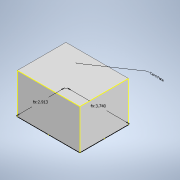
# Autodesk Inventor part: MasterPart
Saved by Autodesk Inventor 2022.2 (Build 262287010, 287A)
## iProperties
Created: 2022-07-12
Part Number: MasterPart
Material: Generic
Document SubType Name: Modeling
Designer: keaton
Density: 1 g/cm^3
Appearance: Default
d0: 3.740 in
d1: 2.913 in
d2: 2.402 in
d3: 0.00 deg
CardWidth: 74.000 mm
CardHeight: 95.000 mm
DeckThickness: 61.000 mm
PlateThickness: 4.000 mm
PuzzleWidth: 15.000 mm
Author: keaton
Autodesk Inventor part; units mm, degrees
ref_plane "YZ Plane" through (0, 0, 0) normal (1, 0, 0) x (0, 1, 0)
ref_plane "XZ Plane" through (0, 0, 0) normal (0, 1, 0) x (-1, 0, 0)
ref_plane "XY Plane" through (0, 0, 0) normal (0, 0, 1) x (1, 0, 0)
sketch "DeckFace" plane through (0, 0, 0) normal (0, 1, 0) x (-1, 0, 0)
  line L0 (-47.5, 37) -> (47.5, 37)
  line L1 (47.5, 37) -> (47.5, -37)
  line L2 (47.5, -37) -> (-47.5, -37)
  line L3 (-47.5, -37) -> (-47.5, 37)
  line L4 (-47.5, 37) -> (47.5, -37) construction
  line L5 (47.5, 37) -> (-47.5, -37) construction
  point P0 (0, 0)
  dimension "d0" = 95
  dimension "d1" = 74
  constraints: 12 end point, 2 midpoint, 2 parallel, 1 horizontal, 1 perpendicular
  measures "d0" distance of L1.end L2.end
  measures "d1" distance of L0.end L1.end
extrude "Extrusion1" add sketch "DeckFace" along normal blind 61
sketch "DeckSide" plane through (-47.5, 0, 37) normal (0, 0, 1) x (1, 0, 0)
  line L0 (0, 61) -> (95, 61) projected
  line L1 (0, 0) -> (0, 61) projected
  line L2 (0, 0) -> (95, 0) projected
  line L3 (95, 0) -> (95, 61) projected
  point P0 (47.5, 0)
sketch "DeckBottom" plane through (47.5, 0, 37) normal (1, 0, 0) x (0, 0, -1)
  line L0 (0, 0) -> (0, 61) projected
  line L1 (0, 61) -> (74, 61) projected
  line L2 (74, 0) -> (74, 61) projected
  line L3 (74, 0) -> (0, 0) projected
  point P0 (37, 0)
equation "\"d0\" = CardHeight"
equation "\"d1\" = CardWidth"
equation "\"d2\" = DeckThickness"
equation "\"CardWidth\" = 74"
equation "\"CardHeight\" = 95"
equation "\"DeckThickness\" = 61"
equation "\"PlateThickness\" = 4"
equation "\"PuzzleWidth\" = 15"
body "Solid1"
